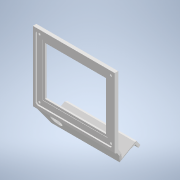
# Autodesk Inventor part: MainHousing_FrontMainShell
Saved by Autodesk Inventor 2021 (Build 250183000, 183)
## iProperties
Created: 2021-04-29
Part Number: MainHousing_FrontMainShell
Material: Generic
Document SubType Name: Modeling
Designer: trent
Density: 1 g/cm^3
Appearance: Default
Author: trent
Autodesk Inventor part; units mm, degrees
ref_plane "YZ Plane" through (0, 0, 0) normal (1, 0, 0) x (0, 1, 0)
ref_plane "XZ Plane" through (0, 0, 0) normal (0, 1, 0) x (-1, 0, 0)
ref_plane "XY Plane" through (0, 0, 0) normal (0, 0, 1) x (1, 0, 0)
sketch "Sketch1" plane through (0, 0, 0) normal (0, 0, 1) x (1, 0, 0)
  line L0 (0, 0) -> (118, 0)
  line L1 (118, 0) -> (118, 100)
  line L2 (118, 100) -> (0, 100)
  line L3 (0, 100) -> (0, 0)
  line L4 (-23.6, 0) -> (141.6, 0) projected
  line L5 (0, -20) -> (0, 120) projected
  dimension "d3" = 118
  dimension "d4" = 100
  dimension "d45" = 0
  dimension "d46" = 0
  constraints: 8 end point, 2 parallel, 1 horizontal, 1 perpendicular
  measures "d3" distance of L1.end L2.end
  measures "d4" distance of L0.end L1.end
  measures "d45" distance between parallel lines of L4 L0
  measures "d46" distance between parallel lines of L5 L3
extrude "Extrusion1" add sketch "Sketch1" along normal blind 5
sketch "Sketch2" plane through (0, 0, 5) normal (0, 0, 1) x (1, 0, 0)
  line L0 (7, 96) -> (111, 96)
  line L1 (114, 93) -> (114, 7)
  line L2 (111, 4) -> (7, 4)
  line L3 (4, 7) -> (4, 93)
  line L4 (118, 100) -> (0, 100) projected
  line L5 (0, 100) -> (0, 0) projected
  line L6 (0, 0) -> (118, 0) projected
  arc A0 (7, 96) -> (4, 93) centre (7, 93) ccw
  arc A1 (114, 93) -> (111, 96) centre (111, 93) ccw
  arc A2 (111, 4) -> (114, 7) centre (111, 7) ccw
  arc A3 (4, 7) -> (7, 4) centre (7, 7) ccw
  point P0 (4, 96)
  point P1 (114, 4)
  point P2 (114, 96)
  dimension "d7" = 110
  dimension "d8" = 92
  dimension "d10" = 4
  dimension "d11" = 4
  dimension "d12" = 3
  constraints: 8 end point, 8 point on circle, 8 tangent, 6 point on line, 4 centre point, 3 equal radius, 2 parallel, 1 horizontal, 1 perpendicular
  measures "d7" distance of point (4, 96) point (114, 96)
  measures "d8" distance of point (114, 96) point (114, 4)
  measures "d10" distance between parallel lines of L5 L3
  measures "d11" distance between parallel lines of L6 L2
  measures "d12" radius of A0
extrude "Extrusion2" cut sketch "Sketch2" against normal blind 2
sketch "Sketch3" plane through (0, 0, 3) normal (0, 0, 1) x (1, 0, 0)
  line L0 (12, 12) -> (106, 12)
  line L1 (106, 12) -> (106, 88)
  line L2 (106, 88) -> (12, 88)
  line L3 (12, 88) -> (12, 12)
  line L4 (7, 96) -> (111, 96) projected
  line L5 (111, 4) -> (7, 4) projected
  line L6 (4, 7) -> (4, 93) projected
  line L7 (114, 93) -> (114, 7) projected
  point P0 (0, 0)
  point P1 (114, 7)
  point P2 (11.024, 100)
  point P3 (121.024, 100)
  point P4 (120, 96)
  point P5 (120, 4)
  dimension "d19" = 8
  dimension "d20" = 8
  dimension "d21" = 8
  dimension "d22" = 8
  constraints: 8 end point, 2 parallel, 1 horizontal, 1 perpendicular, 2 other
  measures "d19" distance between parallel lines of L4 L2
  measures "d20" distance between parallel lines of L5 L0
extrude "Extrusion3" cut sketch "Sketch3" against normal blind 0.5
sketch "Sketch4" plane through (0, 0, 2.5) normal (0, 0, 1) x (1, 0, 0)
  line L0 (15, 85) -> (103, 85)
  line L1 (103, 85) -> (103, 15)
  line L2 (103, 15) -> (15, 15)
  line L3 (15, 15) -> (15, 85)
  line L4 (106, 12) -> (12, 12) projected
  line L5 (12, 12) -> (12, 88) projected
  point P0 (0, 0)
  dimension "d25" = 88
  dimension "d26" = 70
  dimension "d27" = 3
  dimension "d28" = 3
  constraints: 8 end point, 2 parallel, 1 horizontal, 1 perpendicular
  measures "d25" distance of L0.start L0.end
  measures "d26" distance of L2.end L0.start
  measures "d27" distance between parallel lines of L4 L2
  measures "d28" distance between parallel lines of L5 L3
extrude "Extrusion4" cut sketch "Sketch4" against normal through all
sketch "Sketch5" plane through (0, 0, 3) normal (0, 0, 1) x (1, 0, 0)
  circle A0 centre (7.5, 7.5) radius 1.5
  circle A1 centre (110.5, 7.5) radius 1.5
  circle A2 centre (110.5, 92.5) radius 1.5
  circle A3 centre (7.5, 92.5) radius 1.5
  line L0 (7, 96) -> (111, 96) projected
  line L1 (4, 7) -> (4, 93) projected
  line L2 (111, 4) -> (7, 4) projected
  line L3 (114, 93) -> (114, 7) projected
  point P0 (0, 0)
  point P1 (114, 7)
  point P2 (11.024, 100)
  point P3 (121.024, 100)
  point P4 (120, 96)
  point P5 (120, 4)
  dimension "d31" = 3.5
  dimension "d32" = 3.5
  dimension "d33" = 3.5
  dimension "d34" = 3.5
  dimension "d35" = 3.5
  dimension "d36" = 3.5
  dimension "d37" = 3.5
  dimension "d38" = 3.5
  dimension "d39" = 3
  dimension "d40" = 3
  dimension "d41" = 3
  dimension "d42" = 3
  constraints: 4 centre point, 2 other
  measures "d31" distance from line of L0 A3.centre
  measures "d34" distance from line of L2 A0.centre
  measures "d36" distance from line of L2 A1.centre
  measures "d38" distance from line of L0 A2.centre
  measures "d39" diameter of A2
  measures "d40" diameter of A3
  measures "d41" diameter of A0
  measures "d42" diameter of A1
extrude "Extrusion5" cut sketch "Sketch5" against normal blind 3.5
sketch "Sketch6" plane through (0, 0, 0) normal (-1, 0, 0) x (0, 0, 1)
  line L0 (-1, 1) -> (-13.2791, -20.2679)
  line L1 (5, 0) -> (5, 100) projected
  line L2 (1.259, -2.0155) -> (-10.2791, -22)
  line L3 (-13.2791, -20.2679) -> (-10.2791, -22)
  line L4 (-1, 1) -> (0, 1)
  line L5 (0, 0) -> (0, 100) projected
  line L6 (5, 0) -> (4.5, -0.866)
  line L7 (4.5, -0.866) -> (3.25, -0.866)
  line L8 (3.25, -0.866) -> (1.259, -2.0155)
  line L9 (0, 0) -> (5, 0) projected
  line L10 (5, 0) -> (0, 0)
  dimension "d47" = 30
  dimension "d48" = 30
  dimension "d49" = 90
  dimension "d50" = 22
  dimension "d51" = 120
  dimension "d52" = 1
  dimension "d53" = 1.25
  dimension "d54" = 150
  dimension "d55" = 0
  dimension "d57" = 90
  dimension "d58" = 1
  dimension "d59" = 3
  dimension "d60" = 1
  dimension "d67" = 30
  dimension "d68" = 120
  dimension "d69" = 150
  constraints: 16 end point, 3 horizontal, 1 other
  measures "d47" angle of L1 L2
  measures "d48" angle of L0 L1
  measures "d49" angle of L2 L3
  measures "d50" vertical distance of L1.start L2.end
  measures "d51" angle of L0 L4
  measures "d52" distance of L1.start L6.end
  measures "d53" distance of L6.end L7.end
  measures "d54" angle of L8 L7
  measures "d55" distance from line of L5 L4.end
  measures "d57" angle of L3 L0
  measures "d58" distance of L0.start L4.end
  measures "d59" horizontal distance of L0.end L2.end
  measures "d60" distance of L5.start L4.end
  measures "d67" angle of L1 L6
  measures "d68" angle of L7 L6
  measures "d69" angle of L2 L8
extrude "Extrusion6" add sketch "Sketch6" against normal blind 118
sketch "Sketch7" plane through (0, -22, -10.2791) normal (0, -0.5, 0.8660254) x (1, 0, 0)
  line L0 (0, 26.6921) -> (118, 26.6921) projected
  circle A0 centre (25, 13.0581) radius 8
  line L1 (118, 25.0581) -> (0, 25.0581) projected
  line L2 (0, 0) -> (0, 23.0761) projected
  point P0 (0, 24.1921)
  dimension "d70" = 16
  dimension "d71" = 12
  dimension "d72" = 25
  constraints: 1 centre point
  measures "d70" diameter of A0
  measures "d71" distance from line of A0.centre L1
  measures "d72" distance from line of L2 A0.centre
extrude "Extrusion7" cut sketch "Sketch7" against normal up to next
sketch "Sketch8" plane through (0, -22, -10.2791) normal (0, -0.5, 0.8660254) x (1, 0, 0)
  circle A0 centre (25, 13.0581) radius 8 projected
  circle A1 centre (25, 13.0581) radius 11.125
  point P0 (0, 24.1921)
  dimension "d75" = 22.25
  constraints: 1 centre point, 1 coincident
  measures "d75" diameter of A1
extrude "Extrusion8" cut sketch "Sketch8" along normal blind 1
sketch "Sketch9" plane through (0, 100, 0) normal (-1, 0, 0) x (0, 0, 1)
  line L0 (-10.2791, -122) -> (1.259, -102.0155) projected
  line L1 (-10.2791, -122) -> (-11.7791, -124.5981)
  line L2 (-11.7791, -124.5981) -> (-32.7791, -112.4737)
  line L3 (-32.7791, -112.4737) -> (-31.2791, -109.8756)
  line L4 (-1, -99) -> (-13.2791, -120.2679) projected
  line L5 (-31.2791, -109.8756) -> (-13.2791, -120.2679)
  line L6 (-13.2791, -120.2679) -> (-10.2791, -122)
  point P0 (0, -100)
  dimension "d79" = 3
  dimension "d80" = 90
  dimension "d82" = 90
  dimension "d83" = 90
  dimension "d84" = 90
  dimension "d85" = 21
  constraints: 10 end point, 2 perpendicular, 1 collinear
  measures "d79" distance of L0.start L1.end
  measures "d80" angle of L5 L3
  measures "d82" angle of L2 L1
  measures "d83" angle of L4 L5
  measures "d84" angle of L2 L3
  measures "d85" horizontal distance of L1.end L2.end
extrude "Extrusion9" add sketch "Sketch9" against normal blind 118
sketch "Sketch10" plane through (118, 100, 0) normal (1, 0, 0) x (0, 0, -1)
  line L0 (35.9184, -109.7111) -> (41.7463, -118.0342) projected
  line L1 (31.2791, -109.8756) -> (32.7791, -112.4737) projected
  line L2 (41.7463, -118.0342) -> (38.8793, -120.0417)
  line L3 (32.7791, -112.4737) -> (33.3495, -112.1444)
  line L4 (38.8793, -120.0417) -> (33.3495, -112.1444)
  line L5 (31.2791, -109.8756) -> (34.6648, -107.9209)
  line L6 (41.7463, -118.0342) -> (34.6648, -107.9209)
  line L7 (32.7791, -112.4737) -> (11.7791, -124.5981) projected
  point P0 (0, -100)
  dimension "d88" = 3.5
  dimension "d93" = 3.5
  dimension "d97" = 0
  constraints: 10 end point, 1 point on line
  measures "d88" distance of L0.end L2.end
  measures "d93" distance from line of L3.end L0
  measures "d97" distance between parallel lines of L7 L3
extrude "Extrusion10" add sketch "Sketch10" against normal blind 118
fillet "Fillet1" radius 8 1 edges at (59, 1, 0)
chamfer "Chamfer1" distance 2.2 angle 45 1 edges at (59, -7.9209, -34.6648)
chamfer "Chamfer2" distance 2 distance2 8 1 edges at (59, -12.1444, -33.3495) measured on face at (78.6667, -14.7768, -35.1927)
sketch "Sketch11" plane through (25, -10.6913, -3.75) normal (0, -0.5, 0.8660254) x (1, 0, 0)
  line L0 (-25, -16.0581) -> (-25, 10.0179) projected
  line L1 (-25, 10.0179) -> (-25, 4.5179)
  line L2 (-25, 4.5179) -> (-15.4052, -16.0581)
  line L3 (-25, -25.6623) -> (-25, -18.0505) projected
  line L4 (-25, 4.5179) -> (-25, -25.6623)
  line L5 (-25, -25.6623) -> (-15.4052, -25.6623)
  line L6 (-25, -16.0581) -> (93, -16.0581) projected
  line L7 (-15.4052, -16.0581) -> (-15.4052, -25.6623)
  line L8 (93, 10.0179) -> (93, 4.5179)
  line L9 (93, 4.5179) -> (83.4052, -16.0581)
  line L10 (83.4052, -16.0581) -> (83.4052, -25.6623)
  line L11 (93, -25.6623) -> (83.4052, -25.6623)
  line L12 (93, -25.6623) -> (93, 4.5179)
  line L13 (93, 10.0179) -> (93, -16.0581) projected
  point P0 (-25, 11.134)
  point P1 (-25, -18.0505)
  dimension "d101" = 5.5
  dimension "d102" = 25
  dimension "d105" = 5.5
  dimension "d106" = 0
  dimension "d107" = 35.6803
  constraints: 20 end point, 2 collinear, 2 perpendicular, 2 point on line
  measures "d101" distance of L0.end L1.end
  measures "d102" angle of L0 L2
  measures "d105" distance of L8.start L8.end
  measures "d106" distance between parallel lines of L13 L12
  measures "d107" distance of L11.start L8.start
extrude "Extrusion11" cut sketch "Sketch11" against normal through all
equation "\"d39\" = d41"
equation "\"d40\" = d41"
equation "\"d42\" = d41"
body "Solid1"
